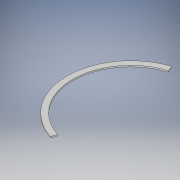
# Autodesk Inventor part: 2AM-17-P-5201 - claw part
Saved by Autodesk Inventor 2017 (Build 210142000, 142)
## iProperties
Created: 2017-12-27
Part Number: 2AM-17-P-5201 - claw part
Material: Generic
Document SubType Name: Modeling
Designer: Micah
Density: 1 g/cm^3
Appearance: Default
Author: Micah
Autodesk Inventor part; units mm, degrees
ref_plane "YZ Plane" through (0, 0, 0) normal (1, 0, 0) x (0, 1, 0)
ref_plane "XZ Plane" through (0, 0, 0) normal (0, 1, 0) x (-1, 0, 0)
ref_plane "XY Plane" through (0, 0, 0) normal (0, 0, 1) x (1, 0, 0)
sketch "Sketch1" plane through (0, 0, 0) normal (0, 1, 0) x (-1, 0, 0)
  arc A0 (0, 132.08) -> (-132.08, 0) centre (0, 0) ccw
  arc A1 (132.08, 0) -> (0, 132.08) centre (0, 0) ccw
  arc A2 (40.815, -125.6155) -> (132.08, 0) centre (0, 0) ccw
  arc A3 (-132.08, 0) -> (-106.855, -77.6347) centre (0, 0) ccw
  arc A4 (44.7395, -137.694) -> (-117.1295, -85.0995) centre (0, 0) ccw
  line L0 (40.815, -125.6155) -> (44.7395, -137.694)
  line L1 (-106.855, -77.6347) -> (-117.1295, -85.0995)
  line L2 (40.815, 125.6155) -> (44.7395, 137.694)
  point P0 (0, 0)
  dimension "d0" = 132.08
  dimension "d1" = 132.08
  dimension "d2" = 132.08
  dimension "d3" = 132.08
  dimension "d4" = 132.08
  dimension "d13" = 289.56
  dimension "d15" = 72
  constraints: 12 point on circle, 6 end point, 5 centre point, 2 concentric
  measures "d0" distance of point (0, 0) A0.end
  measures "d1" distance of point (0, 0) A0.start
  measures "d2" radius of A0
  measures "d3" distance of L1.start A0.centre
  measures "d4" distance of A0.centre A1.start
  measures "d13" diameter of A4
  measures "d15" angle of L1 L0
extrude "Extrusion1" add sketch "Sketch1" along normal blind 3.175 contours L2 A4 L0 A2 A1
body "Solid1"
